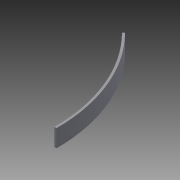
# Autodesk Inventor part: Part13
Saved by Autodesk Inventor 2016 (Build 200138000, 138)
## iProperties
Created: 2016-01-27
Part Number: Part13
Material: Generic
Document SubType Name: Modeling
Designer: 278648
Density: 1 g/cm^3
Appearance: Default
Author: 278648
Autodesk Inventor part; units mm, degrees
ref_plane "YZ Plane" through (0, 0, 0) normal (1, 0, 0) x (0, 1, 0)
ref_plane "XZ Plane" through (0, 0, 0) normal (0, 1, 0) x (-1, 0, 0)
ref_plane "XY Plane" through (0, 0, 0) normal (0, 0, 1) x (1, 0, 0)
sketch "Sketch1" plane through (0, 0, 0) normal (0, 1, 0) x (-1, 0, 0)
  arc A0 (-241.3, 0) -> (-170.6249, -170.6249) centre (0, 0) ccw
  arc A1 (-238.125, 0) -> (-168.3798, -168.3798) centre (0, 0) ccw
  line L0 (-168.3798, -168.3798) -> (-170.6249, -170.6249)
  line L1 (-238.125, 0) -> (-241.3, 0)
  dimension "d0" = 482.6
  dimension "d1" = 3.175
  dimension "d2" = 45
  constraints: 4 end point, 4 point on circle, 2 centre point, 2 coincident, 1 horizontal
  measures "d0" diameter of A0
  measures "d1" radial gap between concentric circles of A0 A1
  measures "d2" angle of L0 L1
extrude "Extrusion1" add sketch "Sketch1" along normal blind 25.4
body "Solid1"
